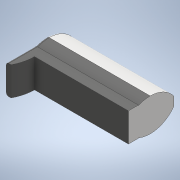
# Autodesk Inventor part: Sci-Fi Raycasting weapon B
Saved by Autodesk Inventor 2020 (Build 240168000, 168)
## iProperties
Created: 2019-09-05
Part Number: Sci-Fi Raycasting weapon B
Material: Generic
Document SubType Name: Modeling
Designer: Victor
Density: 1 g/cm^3
Appearance: Default
Author: Victor
Autodesk Inventor part; units mm, degrees
ref_plane "YZ Plane" through (0, 0, 0) normal (1, 0, 0) x (0, 1, 0)
ref_plane "XZ Plane" through (0, 0, 0) normal (0, 1, 0) x (-1, 0, 0)
ref_plane "XY Plane" through (0, 0, 0) normal (0, 0, 1) x (1, 0, 0)
sketch "Sketch1" plane through (0, 0, 0) normal (0, 0, 1) x (1, 0, 0)
  line L0 (0, 0) -> (-20, 0)
  line L1 (-20, 0) -> (-20, 5)
  line L2 (-20, 5) -> (0, 5)
  line L3 (0, 5) -> (0, 0)
  dimension "d0" = 20
  dimension "d1" = 5
  constraints: 8 end point, 2 parallel, 1 horizontal, 1 perpendicular
  measures "d0" distance of L1.end L2.end
  measures "d1" distance of L0.end L1.end
extrude "Extrusion1" add sketch "Sketch1" along normal blind 7
sketch "Sketch2" plane through (0, 0, 0) normal (1, 0, 0) x (0, 0, -1)
  line L0 (0, 5) -> (-7, 5) projected
  line L1 (-7, 5) -> (-4.5, 5)
  line L2 (0, 5) -> (0, 0) projected
  line L3 (0, 5) -> (-2.5, 5)
  arc A0 (-4.5, 5) -> (-7, 0) centre (-0.7528, 0.0014) ccw
  arc A1 (0, 0) -> (-2.5, 5) centre (-6.2429, 0.0035) ccw
  line L4 (-7, 0) -> (-7, 5) projected
  line L5 (-7, 5) -> (-7, 0.0014)
  line L6 (0, 5) -> (0, 0)
  dimension "d4" = 2.5
  dimension "d5" = 2.5
  dimension "d6" = 6.2472
  dimension "d7" = 6.2429
  dimension "d10" = 5
  constraints: 8 end point, 5 point on circle, 3 point on line, 2 centre point
  measures "d4" distance of L0.end L1.end
  measures "d5" distance of L0.start L3.end
  measures "d6" radius of A0
  measures "d7" radius of A1
  measures "d10" distance from line of L2.end L0
extrude "Extrusion3" cut sketch "Sketch2" against normal blind 22
sketch "Sketch3" plane through (-20, 0, 7) normal (0, -1, 0) x (1, 0, 0)
  line L0 (20, -7) -> (20, 0) projected
  line L1 (20, -7) -> (0, -7) projected
  line L2 (20, 0) -> (0, 0)
  line L3 (0, 0) -> (0, -7)
  line L4 (0, -7) -> (20, -7)
  line L5 (20, -7) -> (20, 0)
  constraints: 8 end point, 2 parallel, 1 horizontal, 1 perpendicular
extrude "Extrusion4" add sketch "Sketch3" along normal blind 4.636
sketch "Sketch6" plane through (0, 5, 4.5) normal (1, 0, 0) x (0, 0, -1)
  line L0 (-2.5, -4.9986) -> (-2.5, -9.636) projected
  line L1 (-2.5, -9.636) -> (-0.5, -9.636)
  line L2 (4.5, -9.636) -> (-2.5, -9.636) projected
  line L3 (4.5, -9.636) -> (2.5, -9.636)
  arc A0 (-2.5, -4.9986) -> (-0.5, -9.636) centre (3.8682, -5.0021) ccw
  line L4 (4.5, -5) -> (4.5, -9.636) projected
  arc A1 (2.5, -9.636) -> (4.5, -5) centre (-1.8727, -5.0002) ccw
  dimension "d36" = 2
  dimension "d37" = 2
  constraints: 4 end point, 4 point on circle, 2 centre point, 2 point on line
  measures "d36" distance of L0.end L1.end
  measures "d37" distance of L2.start L3.end
extrude "Extrusion9" cut sketch "Sketch6" against normal blind 25
sketch "Sketch7" plane through (-20, 5, 2.5) normal (-1, 0, 0) x (0, 0, 1)
  line L0 (2.5, -9.636) -> (-0.5, -9.636) projected
  line L1 (1, -7.511) -> (4.065, -7.511)
  line L2 (4.065, -7.511) -> (4.065, -9.636)
  line L3 (4.065, -9.636) -> (1, -9.636)
  line L4 (1, -9.636) -> (1, -7.511)
  line L5 (1, -7.511) -> (-2.056, -7.511)
  line L6 (-2.056, -7.511) -> (-2.056, -9.636)
  line L7 (-2.056, -9.636) -> (1, -9.636)
  line L8 (1, -9.636) -> (1, -7.511)
  point P0 (-2.5, -5)
  dimension "d40" = 2.125
  dimension "d41" = 3.5
  dimension "d42" = 3.065
  dimension "d43" = 3.056
  constraints: 16 end point, 4 parallel, 2 horizontal, 2 perpendicular, 2 point on line
  measures "d40" distance from line of L0 L1.start
  measures "d41" horizontal distance of L1.start point (-2.5, -5)
  measures "d42" distance of L2.end L3.end
  measures "d43" distance of L7.end L6.end
extrude "Extrusion10" add sketch "Sketch7" against normal blind 20
sketch "Sketch8" plane through (-20, 5, 2.5) normal (-1, 0, 0) x (0, 0, 1)
  line L0 (0, 0) -> (2, 0) projected
  arc A0 (0, 0) -> (-2.5, -5) centre (3.7429, -4.9965) ccw
  arc A1 (4.5, -4.9986) -> (2, 0) centre (-1.7472, -4.9986) ccw projected
  arc A2 (4.5, -4.9986) -> (2, 0) centre (-1.7472, -4.9986) ccw
  arc A3 (0, 0) -> (-2.5, -5) centre (3.7429, -4.9965) ccw projected
  line L1 (0, 0) -> (2, 0)
  line L2 (-2.056, -9.636) -> (-2.056, -7.511) projected
  line L3 (-2.056, -7.511) -> (-2.056, -9.636)
  line L4 (-2.056, -9.636) -> (4.065, -9.636)
  line L5 (4.065, -7.511) -> (4.065, -9.636) projected
  line L6 (4.065, -9.636) -> (4.065, -7.511)
  line L7 (3.985, -7.511) -> (4.065, -7.511) projected
  line L8 (4.065, -7.511) -> (3.985, -7.511)
  line L9 (-1.9845, -7.511) -> (-2.056, -7.511) projected
  line L10 (-1.9845, -7.511) -> (-2.056, -7.511)
  arc A4 (3.985, -7.511) -> (4.5, -4.9986) centre (-1.8682, -5.0021) ccw projected
  arc A5 (3.985, -7.511) -> (4.5, -4.9986) centre (-1.8682, -5.0021) ccw
  arc A6 (-2.5, -5) -> (-1.9845, -7.511) centre (3.8727, -5.0002) ccw projected
  arc A7 (-2.5, -5) -> (-1.9845, -7.511) centre (3.8727, -5.0002) ccw
  line L11 (4.065, -9.636) -> (-2.056, -9.636) projected
  line L12 (4.065, -9.636) -> (4.065, -13.636)
  line L13 (4.065, -13.636) -> (-2.056, -13.636)
  line L14 (-2.056, -13.636) -> (-2.056, -9.636)
  dimension "d46" = 4
  constraints: 18 end point, 8 point on circle, 4 centre point, 4 perpendicular, 3 collinear, 2 vertical
  measures "d46" distance of L4.end L12.end
extrude "Extrusion11" add sketch "Sketch8" along normal blind 2
sketch "Sketch9" plane through (0, -4.636, 6.565) normal (0, 0, 1) x (1, 0, 0)
  line L0 (-20, -4) -> (-22, -4) projected
  line L1 (-20, 0) -> (0, 0) projected
  arc A0 (-21, -4) -> (-20, 0) centre (-28.3129, -0.0468) ccw
  line L2 (-21, -4) -> (-20, -4)
  line L3 (-20, -4) -> (-20, 0) projected
  line L4 (-20, -4) -> (-20, 0)
  point P0 (0, 4.636)
  point P1 (-20, -0.0935)
  constraints: 4 end point, 2 collinear, 2 point on circle, 1 centre point, 1 midpoint
extrude "Extrusion12" cut sketch "Sketch9" against normal blind 10
fillet "Fillet1" radius 0.5 6 edges at (-22, -1.281, 6.8703) (-22, 2.7959, 6.3402) (-22, -5.5735, 6.565) (-22, 2.7955, 0.6591) (-22, -1.2817, 0.1302) (-22, -5.5735, 0.444)
body "Solid1"
